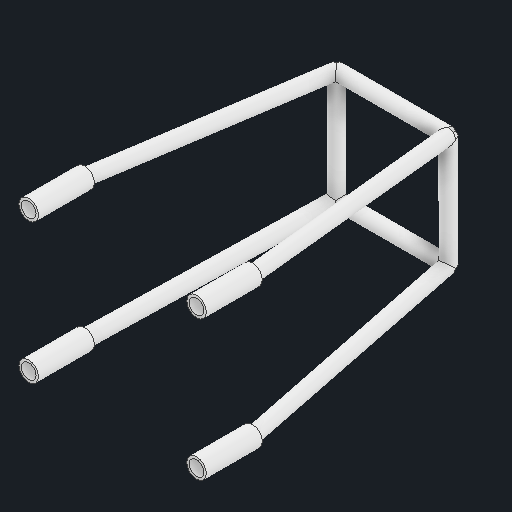
# Autodesk Inventor part: RCPlaneSkeletonFront1
Saved by Autodesk Inventor 2026.1 (Build 301233000, 233)
## iProperties
Created: 2026-02-24
Part Number: RCPlaneSkeletonFront1
Material: PC/ABS Plastic
Document SubType Name: Modeling
Designer: morri
Density: 1.1 g/cm^3
Appearance: Smooth - White
Mass: 12.2786 g
Surface Area: 104.353 cm^2
Volume: 11.1624 cm^3
Author: morri
Autodesk Inventor part; units mm, degrees
sketch "Sketch1" plane through (0, 0, 0) normal (0, 0, 1) x (1, 0, 0)
  circle A0 centre (0, 0) radius 3.5
  circle A1 centre (0, 50) radius 3.5
  circle A2 centre (60, 0) radius 3.5
  circle A3 centre (60, 50) radius 3.5
  dimension "d2" = 7
  dimension "d3" = 7
  dimension "d4" = 7
  dimension "d5" = 7
  constraints: 4 centre point, 1 coincident
  measures "d2" diameter of A0
  measures "d3" diameter of A1
  measures "d4" diameter of A2
  measures "d5" diameter of A3
extrude "Extrusion1" add sketch "Sketch1" along normal blind 20
sketch "Sketch2" plane through (0, 0, 20) normal (0, 0, 1) x (1, 0, 0)
  circle A0 centre (0, 0) radius 3.5 projected
  circle A1 centre (0, 0) radius 2.65
  circle A2 centre (0, 50) radius 3.5 projected
  circle A3 centre (0, 50) radius 2.65
  circle A4 centre (60, 50) radius 3.5 projected
  circle A5 centre (60, 50) radius 2.65
  circle A6 centre (60, 0) radius 3.5 projected
  circle A7 centre (60, 0) radius 2.65
  dimension "d8" = 5.3
  dimension "d9" = 5.3
  dimension "d10" = 5.3
  dimension "d11" = 5.3
  constraints: 4 centre point, 4 coincident
  measures "d8" diameter of A1
  measures "d9" diameter of A3
  measures "d10" diameter of A5
  measures "d11" diameter of A7
extrude "Extrusion2" cut sketch "Sketch2" against normal blind 15 contours A1 | A3 | A5 | A7
sketch "Sketch4" plane through (0, 0, 0) normal (1, 0, 0) x (0, 1, 0)
  point P0 (0, 0)
ref_plane "Work Plane1" through (0, 0, -80) normal (0, 0, -1) x (-1, 0, 0)
sketch "Sketch5" plane through (0, 0, -80) normal (0, 0, -1) x (-1, 0, 0)
  circle A0 centre (-10, 47.9375) radius 2.5
  circle A1 centre (-50, 47.9375) radius 2.5
  circle A2 centre (-50, 7.9375) radius 2.5
  circle A3 centre (-10, 7.9375) radius 2.5
  point P0 (0, 0)
  dimension "d20" = 5
  dimension "d21" = 5
  dimension "d22" = 5
  dimension "d23" = 5
  constraints: 4 centre point
  measures "d20" diameter of A0
  measures "d21" diameter of A1
  measures "d22" diameter of A2
  measures "d23" diameter of A3
sketch "Sketch6" plane through (0, 0, 0) normal (0, 0, 1) x (1, 0, 0)
  circle A0 centre (0, 0) radius 2.65 projected
  circle A1 centre (0, 0) radius 2.5
  circle A2 centre (0, 50) radius 2.65 projected
  circle A3 centre (0, 50) radius 2.5
  circle A4 centre (60.325, 50) radius 2.5
  circle A5 centre (60, 0) radius 2.65 projected
  circle A6 centre (60, 0) radius 2.5
  dimension "d24" = 5
  dimension "d25" = 5
  dimension "d26" = 5
  dimension "d27" = 5
  constraints: 4 centre point, 3 coincident
  measures "d24" diameter of A1
  measures "d25" diameter of A3
  measures "d26" diameter of A4
  measures "d27" diameter of A6
sketch3d "3D Sketch1"
  line L0 (0, 0, 0) -> (10, 7.9375, -80)
sweep "Sweep1" add profiles "Sketch6" path "3D Sketch1" contours A0 | A1
sketch "Sketch7" plane through (0, 0, 0) normal (0, 0, 1) x (1, 0, 0)
  circle A0 centre (0, 50) radius 2.65 projected
  circle A1 centre (0, 50) radius 2.5
  point P0 (0, 0)
  dimension "d30" = 5
  constraints: 1 centre point, 1 coincident
  measures "d30" diameter of A1
sketch3d "3D Sketch2"
  line L0 (0, 50, 0) -> (10, 47.9375, -80)
sweep "Sweep2" add profiles "Sketch7" path "3D Sketch2" contours A1
sketch "Sketch8" plane through (0, 0, 0) normal (0, 0, 1) x (1, 0, 0)
  circle A0 centre (60, 50) radius 3.5 projected
  circle A1 centre (60, 50) radius 2.5
  point P0 (0, 0)
  dimension "d33" = 5
  constraints: 1 centre point, 1 coincident
  measures "d33" diameter of A1
sketch "Sketch9" plane through (60, 0, 0) normal (0, 0, -1) x (-1, 0, 0)
  circle A0 centre (0, 0) radius 3.5 projected
  circle A1 centre (0, 0) radius 2.5
  point P0 (60, 0)
  dimension "d34" = 5
  constraints: 1 centre point, 1 coincident
  measures "d34" diameter of A1
sketch3d "3D Sketch3"
  line L0 (60, 50, 0) -> (50, 47.9375, -80)
sweep "Sweep3" add profiles "Sketch8" path "3D Sketch3" contours A1
sketch3d "3D Sketch4"
  line L0 (60, 0, 0) -> (50, 7.9375, -80)
sweep "Sweep4" add profiles "Sketch9" path "3D Sketch4" contours A1
ref_plane "Work Plane3" through (10, 47.9375, -80) normal (1, 0, 0) x (0, 1, 0)
sketch "Sketch10" plane through (10, 47.9375, -80) normal (1, 0, 0) x (0, 1, 0)
  circle A0 centre (0, 0) radius 2.5
  circle A1 centre (-40, 0) radius 2.5
  point P0 (-47.9375, 80)
  dimension "d39" = 5
  dimension "d40" = 5
  constraints: 2 centre point
  measures "d39" diameter of A0
  measures "d40" diameter of A1
extrude "Extrusion3" add sketch "Sketch10" along normal blind 40
ref_plane "Work Plane5" through (52.5, 47.9375, -80) normal (0, 1, 0) x (-1, 0, 0)
sketch "Sketch12" plane through (52.5, 47.9375, -80) normal (0, 1, 0) x (-1, 0, 0)
  line L0 (2.5, 0.1309) -> (2.5, 0) projected
  circle A0 centre (2.5, 0) radius 2.5
  line L1 (42.5, 0) -> (45, 0) projected
  circle A1 centre (42.5, 0) radius 2.5
  point P0 (52.5, 80)
  dimension "d46" = 5
  dimension "d47" = 5
  constraints: 2 centre point
  measures "d46" diameter of A0
  measures "d47" diameter of A1
extrude "Extrusion4" add sketch "Sketch12" against normal blind 40
equation "\"ConnectTol\" = 0.3"
body "Solid1"
